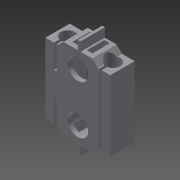
# Autodesk Inventor part: XCarriageV8
Saved by Autodesk Inventor 2015 (Build 190159000, 159)
## iProperties
Created: 2014-08-21
Part Number: XCarriageV8
Material: Generic
Document SubType Name: Modeling
Designer: t_clevj
Density: 1 g/cm^3
Appearance: Default
Author: t_clevj
Autodesk Inventor part; units mm, degrees
ref_plane "YZ Plane" through (0, 0, 0) normal (1, 0, 0) x (0, 1, 0)
ref_plane "XZ Plane" through (0, 0, 0) normal (0, 1, 0) x (-1, 0, 0)
ref_plane "XY Plane" through (0, 0, 0) normal (0, 0, 1) x (1, 0, 0)
sketch "Sketch1" plane through (0, 0, 0) normal (0, 0, 1) x (1, 0, 0)
  circle A0 centre (0, 0) radius 8
  circle A1 centre (50, 0) radius 8
  line L0 (-1.5, -7.8581) -> (-1.5, -14)
  line L1 (-1.5, -14) -> (-11, -14)
  line L2 (-11, -14) -> (-11, 13)
  line L3 (-11, 13) -> (61, 13)
  line L4 (61, 13) -> (61, -14)
  line L5 (61, -14) -> (51.5, -14)
  line L6 (51.5, -14) -> (51.5, -7.8581)
  line L7 (1.5, -7.8581) -> (1.5, -14)
  line L8 (1.5, -14) -> (48.5, -14)
  line L9 (48.5, -14) -> (48.5, -7.8581)
  dimension "d0" = 16
  dimension "d1" = 16
  dimension "d2" = 50
  dimension "d3" = 1.5
  dimension "d4" = 1.5
  dimension "d7" = 11
  dimension "d8" = 11
  dimension "d9" = 1.5
  dimension "d10" = 1.5
  dimension "d29" = 27
  dimension "d30" = 14
  constraints: 20 end point, 6 perpendicular, 4 point on circle, 2 centre point, 2 horizontal alignment, 2 point on line, 2 vertical, 1 coincident, 1 horizontal
  measures "d0" diameter of A0
  measures "d1" diameter of A1
  measures "d2" distance of point (0, 0) A1.centre
  measures "d3" distance from line of A1.centre L6
  measures "d4" distance from line of point (0, 0) L0
  measures "d7" distance from line of point (0, 0) L2
  measures "d8" distance from line of L4 A1.centre
  measures "d9" distance from line of point (0, 0) L7
  measures "d10" distance from line of A1.centre L9
  measures "d29" distance of L1.end L2.end
  measures "d30" distance from line of point (0, 0) L8
extrude "Extrusion1" add sketch "Sketch1" along normal blind 90 contours A0 L0 L1 L2 L3 L4 L5 L6 A1 L9 L8 L7
sketch "Sketch2" plane through (-11, 13, 0) normal (0, 1, 0) x (1, 0, 0)
  line L0 (0, 0) -> (0, -90) projected
  line L1 (72, -90) -> (0, -90) projected
  circle A0 centre (36, -18) radius 13.3
  circle A1 centre (36, -72) radius 13.3
  point P0 (11, 0)
  dimension "d13" = 26.6
  dimension "d14" = 26.6
  dimension "d15" = 54
  dimension "d16" = 18
  dimension "d17" = 36
  constraints: 2 centre point, 1 vertical alignment
  measures "d13" diameter of A0
  measures "d14" diameter of A1
  measures "d15" distance of A0.centre A1.centre
  measures "d16" distance from line of L1 A1.centre
  measures "d17" distance from line of L0 A1.centre
extrude "Extrusion2" cut sketch "Sketch2" against normal up to surface (27 mm away)
sketch "Sketch3" plane through (-11, 13, 0) normal (0, 1, 0) x (1, 0, 0)
  line L0 (72, 0) -> (0, 0) projected
  line L1 (0, 0) -> (0, -90) projected
  line L2 (72, -90) -> (0, -90) projected
  line L3 (72, 0) -> (72, -90) projected
  line L4 (12.5, 0) -> (59.5, 0) projected
  line L5 (20, 0) -> (20, -6)
  line L6 (52, 0) -> (52, -6)
  line L7 (20, -90) -> (20, -84)
  line L8 (52, -90) -> (52, -84)
  line L9 (52, -84) -> (72, -84)
  line L10 (20, -84) -> (0, -84)
  line L11 (0, 0) -> (0, -90) projected
  line L12 (20, -6) -> (0, -6)
  line L13 (52, -6) -> (72, -6)
  line L14 (0, -6) -> (0, 0)
  line L15 (0, 0) -> (20, 0)
  point P0 (11, 0)
  dimension "d20" = 32
  dimension "d21" = 20
  dimension "d22" = 78
  dimension "d23" = 6
  constraints: 20 end point, 8 point on line, 7 perpendicular, 2 collinear, 2 horizontal alignment, 2 vertical alignment, 1 horizontal
  measures "d20" distance of L6.start L5.start
  measures "d21" distance of L0.end L5.start
  measures "d22" distance between parallel lines of L9 L13
  measures "d23" distance between parallel lines of L0 L12
extrude "Extrusion3" cut sketch "Sketch3" against normal up to surface (27 mm away) contours L3 L13 L6 L0 | L3 L2 L8 L9 | L5 L12 L1 L0 | L2 L1 L10 L7
chamfer "Chamfer1" distance 6 angle 45 4 edges at (9, -0.5, 84) (41, -0.5, 84) (41, -0.5, 6) (9, -0.5, 6)
sketch "Sketch4" plane through (1.5, -14, 6) normal (0, -1, 0) x (1, 0, 0)
  circle A0 centre (23.5, 66) radius 13.3 projected
  circle A1 centre (23.5, 12) radius 13.3 projected
  circle A2 centre (23.5, 66) radius 11.5
  circle A3 centre (23.5, 12) radius 11.5
  point P0 (-1.5, -6)
  dimension "d31" = 23
  dimension "d32" = 23
  constraints: 2 centre point, 2 coincident
  measures "d31" diameter of A2
  measures "d32" diameter of A3
extrude "Extrusion4" add sketch "Sketch4" against normal blind 5
sketch "Sketch6" plane through (61, 13, 84) normal (0, 1, 0) x (1, 0, 0)
  circle A0 centre (-36, 66) radius 13.3 projected
  circle A1 centre (-36, 12) radius 13.3 projected
  line L0 (-49.3, 12) -> (-49.3, 66)
  line L1 (-22.7, 66) -> (-22.7, 12)
  point P0 (-61, 84)
  constraints: 4 end point, 4 point on circle, 3 tangent, 1 parallel
extrude "Extrusion6" cut sketch "Sketch6" against normal up to surface (22 mm away) contours L1 A1 L0 A0
sketch "Sketch5" plane through (61, 13, 84) normal (0, 1, 0) x (1, 0, 0)
  line L0 (0, 78) -> (0, 0) projected
  line L1 (-20, 84) -> (-52, 84) projected
  line L2 (-72, 78) -> (-72, 0) projected
  circle A0 centre (-51, 39) radius 13
  circle A1 centre (-21, 39) radius 13
  point P0 (-61, 84)
  dimension "d35" = 21
  dimension "d36" = 21
  dimension "d37" = 26
  dimension "d38" = 45
  constraints: 2 centre point, 1 equal radius, 1 horizontal alignment
  measures "d35" distance from line of L0 A1.centre
  measures "d36" distance from line of L2 A0.centre
  measures "d37" diameter of A0
  measures "d38" distance from line of L1 A0.centre
extrude "Extrusion5" cut sketch "Sketch5" against normal blind 4
sketch "Sketch7" plane through (1.5, -9, 6) normal (0, 1, 0) x (1, 0, 0)
  arc A0 (10.2, -66) -> (36.8, -66) centre (23.5, -66) ccw projected
  line L0 (36.8, -12) -> (36.8, -66) projected
  line L1 (10.2, -66) -> (10.2, -12) projected
  line L2 (10.2, -26.1116) -> (10.2, -51.8884) projected
  arc A1 (10.2, -26.1116) -> (10.2, -51.8884) centre (8.5, -39) ccw projected
  line L3 (36.8, -51.8884) -> (36.8, -26.1116) projected
  arc A2 (36.8, -51.8884) -> (36.8, -26.1116) centre (38.5, -39) ccw projected
  circle A3 centre (23.5, -12) radius 11.5 projected
  circle A4 centre (23.5, -66) radius 11.5 projected
  arc A5 (21.5, -39) -> (10.2, -26.1116) centre (8.5, -39) ccw
  arc A6 (25.5, -39) -> (36.8, -51.8884) centre (38.5, -39) ccw
  arc A7 (10.2, -66) -> (36.8, -66) centre (23.5, -66) ccw projected
  arc A8 (21.5, -39) -> (29.7641, -53.5837) centre (38.5, -39) ccw
  arc A9 (36.8, -66) -> (29.7641, -53.5837) centre (22.3265, -66) ccw
  arc A10 (25.5, -39) -> (17.2359, -24.4163) centre (8.5, -39) ccw
  arc A11 (10.2, -12) -> (17.2359, -24.4163) centre (24.6735, -12) ccw
  line L4 (36.8, -66) -> (36.8, -51.8884)
  line L5 (10.2, -26.1116) -> (10.2, -12)
  point P0 (-1.5, 6)
  constraints: 12 point on circle, 12 tangent, 6 centre point, 4 coincident, 4 end point, 2 collinear, 2 horizontal alignment
extrude "Extrusion7" add sketch "Sketch7" along normal up to surface (22 mm away) contours A9 A8 A5 L1 A11 A10 A6 L0
sketch "Sketch9" plane through (0, 0, 0) normal (0, 0, -1) x (-1, 0, 0)
  line L0 (-41, 13) -> (-9, 13) projected
  line L1 (-41, 13) -> (-41, -14) projected
  line L2 (-9, -14) -> (-41, -14) construction
  line L3 (-28, -14) -> (-25, -14) construction
  line L4 (-25, -14) -> (-25, 13) construction
  line L5 (-25, 13) -> (-28, 13) construction
  line L6 (-28, 13) -> (-28, -14) construction
  line L7 (-36, -9) -> (-30, -9)
  line L8 (-30, -9) -> (-30, 10.5)
  line L9 (-30, 10.5) -> (-36, 10.5)
  line L10 (-36, 10.5) -> (-36, -9)
  line L11 (-20, 10.5) -> (-14, 10.5)
  line L12 (-14, 10.5) -> (-14, -9)
  line L13 (-14, -9) -> (-20, -9)
  line L14 (-20, -9) -> (-20, 10.5)
  line L15 (-22, 13) -> (-22, -14) construction
  point P0 (0, 0)
  dimension "d66" = 3
  dimension "d67" = 16
  dimension "d68" = 6
  dimension "d69" = 19.5
  dimension "d70" = 3
  dimension "d71" = 2
  dimension "d72" = 2
  dimension "d73" = 2.5
  dimension "d74" = 2.5
  constraints: 26 end point, 6 parallel, 3 horizontal, 3 perpendicular, 3 point on line, 2 equal length, 1 midpoint, 1 vertical
  measures "d66" distance between parallel lines of L4 L6
  measures "d67" distance between parallel lines of L1 L4
  measures "d68" distance of L8.end L9.end
  measures "d69" distance of L9.end L7.start
  measures "d70" distance between parallel lines of L15 L4
  measures "d71" distance between parallel lines of L6 L8
  measures "d72" distance between parallel lines of L15 L14
  measures "d73" distance between parallel lines of L0 L11
  measures "d74" distance between parallel lines of L0 L9
extrude "Extrusion8" cut sketch "Sketch9" against normal blind 11.5
sketch "Sketch10" plane through (0, 0, 90) normal (0, 0, 1) x (1, 0, 0)
  line L0 (20, -9) -> (20, 10.5) projected
  line L1 (20, 10.5) -> (14, 10.5) projected
  line L2 (14, 10.5) -> (14, -9) projected
  line L3 (14, -9) -> (20, -9) projected
  line L4 (30, 10.5) -> (30, -9) projected
  line L5 (30, -9) -> (36, -9) projected
  line L6 (36, -9) -> (36, 10.5) projected
  line L7 (36, 10.5) -> (30, 10.5) projected
  point P0 (0, 0)
extrude "Extrusion9" cut sketch "Sketch10" against normal blind 11.5
sketch "Sketch11" plane through (0, 0, 0) normal (0, 0, -1) x (-1, 0, 0)
  line L0 (-41, 13) -> (-9, 13) projected
  line L1 (-9, -14) -> (-41, -14) projected
  line L2 (-25, 13) -> (-28, 13)
  line L3 (-28, 13) -> (-28, -14)
  line L4 (-28, -14) -> (-25, -14)
  line L5 (-25, -14) -> (-25, 13)
  point P0 (0, 0)
  dimension "d85" = 3
  constraints: 8 end point, 2 parallel, 1 horizontal, 1 midpoint, 1 perpendicular, 1 point on line
  measures "d85" distance between parallel lines of L3 L5
extrude "Extrusion10" add sketch "Sketch11" along normal blind 10
sketch "Sketch12" plane through (0, 0, 90) normal (0, 0, 1) x (1, 0, 0)
  line L0 (25, 13) -> (28, 13) projected
  line L1 (28, 13) -> (28, -14) projected
  line L2 (28, -14) -> (25, -14) projected
  line L3 (25, -14) -> (25, 13) projected
  point P0 (0, 0)
extrude "Extrusion11" add sketch "Sketch12" along normal blind 10
sketch "Sketch13" plane through (61, 13, 84) normal (0, 1, 0) x (1, 0, 0)
  arc A0 (-38, 39) -> (-29.7359, 24.4163) centre (-21, 39) ccw projected
  arc A1 (-34, 39) -> (-22.7, 51.8884) centre (-21, 39) ccw projected
  arc A2 (-34, 39) -> (-42.2641, 53.5837) centre (-51, 39) ccw projected
  circle A3 centre (-63, 27) radius 1.5
  circle A4 centre (-63, 51) radius 1.5
  circle A5 centre (-9, 27) radius 1.5
  circle A6 centre (-9, 51) radius 1.5
  point P0 (-11.6358, 48.0173)
  point P1 (-61, 84)
  dimension "d94" = 3
  dimension "d95" = 3
  dimension "d96" = 3
  dimension "d97" = 3
  dimension "d98" = 24
  dimension "d99" = 12
  dimension "d100" = 12
  dimension "d101" = 12
  constraints: 4 centre point, 2 horizontal alignment, 2 vertical alignment
  measures "d94" diameter of A3
  measures "d95" diameter of A4
  measures "d96" diameter of A5
  measures "d97" diameter of A6
  measures "d98" distance of A6.centre A5.centre
  measures "d99" horizontal distance of A0.centre A5.centre
  measures "d100" horizontal distance of A1.centre A5.centre
  measures "d101" horizontal distance of A2.centre A4.centre
extrude "Extrusion12" cut sketch "Sketch13" against normal blind 7.5
ref_plane "Work Plane1" through (-11, -14, 58) normal (0, 0, 1) x (1, 0, 0)
ref_plane "Work Plane2" through (-1.5, -14, 32) normal (0, 0, -1) x (-1, 0, 0)
sketch "Sketch14" plane through (-11, -14, 58) normal (0, 0, 1) x (1, 0, 0)
  line L0 (14, 27) -> (14, 21.4162) projected
  line L1 (0, 27) -> (14, 27) projected
  line L2 (0, 0) -> (0, 27) projected
  line L3 (9.5, 0) -> (0, 0) projected
  line L4 (9.5, 6.1419) -> (9.5, 0) projected
  arc A0 (14, 21.4162) -> (9.5, 6.1419) centre (11, 14) ccw projected
  line L5 (9.5, 6.1419) -> (9.5, 0)
  line L6 (9.5, 0) -> (12.5, 0)
  line L7 (12.5, 0) -> (12.5, 6.1419)
  arc A1 (12.5, 6.1419) -> (9.5, 6.1419) centre (11, 14) ccw
  constraints: 6 end point, 2 perpendicular, 2 point on circle, 1 centre point, 1 coincident, 1 collinear
extrude "Extrusion14" add sketch "Sketch14" against normal up to surface (26 mm away) contours A1 L7 L6 L4 A0
body "Solid1"
